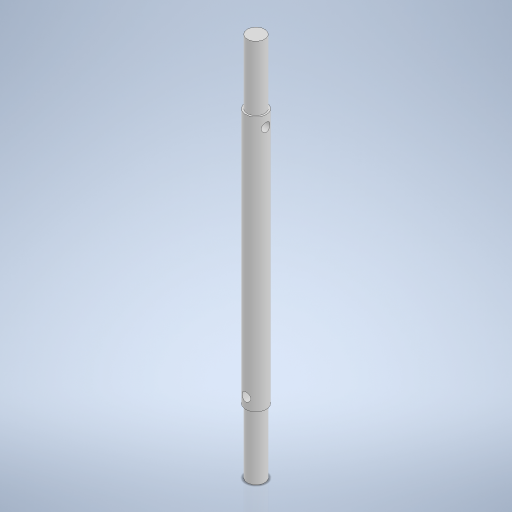
# Autodesk Inventor part: 2011
Saved by Autodesk Inventor 2024 (Build 280153000, 153)
## iProperties
Created: 2024-06-11
Part Number: 2011
Material: Generisch
Document SubType Name: Modeling
Designer: ffogue
Density: 1 g/cm^3
Appearance: Vorgabe
Author: ffogue
Autodesk Inventor part; units mm, degrees
ref_plane "XY Plane" through (0, 0, 0) normal (0, 0, 1) x (1, 0, 0)
sketch "Skizze1" plane through (0, 0, 0) normal (0, 1, 0) x (-1, 0, 0)
  line L0 (0, 0) -> (8, 0)
  line L1 (8, 0) -> (8, -59)
  line L2 (8, -59) -> (9.5, -59)
  line L3 (9.5, -59) -> (9.5, -293)
  line L4 (9.5, -293) -> (8, -293)
  line L5 (8, -293) -> (8, -352)
  line L6 (8, -352) -> (0, -352)
  line L7 (0, -352) -> (0, 0)
  dimension "d0" = 16
  dimension "d1" = 59
  dimension "d2" = 59
  dimension "d3" = 352
  dimension "d4" = 19
  constraints: 16 end point, 6 perpendicular, 2 point on line, 1 horizontal
  measures "d0" diameter of L1 L7
  measures "d1" distance between parallel lines of L0 L2
  measures "d2" distance between parallel lines of L6 L4
  measures "d3" distance between parallel lines of L6 L0
  measures "d4" diameter of L3 L7
revolve "Umdrehung1" add sketch "Skizze1" angle 360 about axis through (0, 0, -352) along (0, 0, 1)
ref_plane "Arbeitsebene1" through (9.5, 0, 0) normal (1, 0, 0) x (0, 1, 0)
sketch "Skizze2" plane through (9.5, 0, 0) normal (1, 0, 0) x (0, 1, 0)
  line L0 (8, 0) -> (-8, 0) projected
  point P0 (0, 0)
  point P1 (0, -69)
  point P2 (0, 0)
  dimension "d7" = 69
  constraints: 1 midpoint, 1 vertical alignment
  measures "d7" distance from line of point (0, -69) L0
hole "Bohrung1" at (9.5, 0, -69) direction (-1, 0, 0) diameter 8 end through all
ref_plane "Arbeitsebene2" through (0, 9.5, 0) normal (0, 1, 0) x (-1, 0, 0)
sketch "Skizze3" plane through (0, 9.5, 0) normal (0, 1, 0) x (-1, 0, 0)
  line L0 (9.5, -293) -> (-9.5, -293) projected
  point P0 (0, 0)
  point P1 (0, -283)
  dimension "d16" = 10
  constraints: 1 vertical alignment
  measures "d16" distance from line of L0 point (0, -283)
hole "Bohrung2" at (0, 9.5, -283) direction (0, -1, 0) diameter 8 end through all
